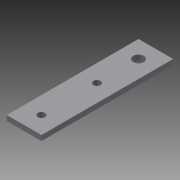
# Autodesk Inventor part: servo catch front c
Saved by Autodesk Inventor 2015 (Build 190159000, 159)
## iProperties
Created: 2015-06-24
Part Number: servo catch front c
Material: 一般
Document SubType Name: Modeling
Designer: kenta
Density: 1 g/cm^3
Appearance: 既定
Author: kenta
Autodesk Inventor part; units mm, degrees
ref_plane "YZ Plane" through (0, 0, 0) normal (1, 0, 0) x (0, 1, 0)
ref_plane "XZ Plane" through (0, 0, 0) normal (0, 1, 0) x (-1, 0, 0)
ref_plane "XY Plane" through (0, 0, 0) normal (0, 0, 1) x (1, 0, 0)
sketch "スケッチ1" plane through (0, 0, 0) normal (0, 0, 1) x (1, 0, 0)
  line L0 (-5, 19) -> (5, 19)
  line L1 (5, 19) -> (5, -19)
  line L2 (5, -19) -> (-5, -19)
  line L3 (-5, -19) -> (-5, 19)
  line L4 (-5, 19) -> (5, -19) construction
  line L5 (5, 19) -> (-5, -19) construction
  point P0 (0, 0)
  dimension "d0" = 10
  dimension "d1" = 38
  constraints: 12 end point, 2 midpoint, 2 parallel, 1 horizontal, 1 perpendicular
  measures "d0" distance of L1.end L2.end
  measures "d1" distance of L0.end L1.end
extrude "押し出し1" add sketch "スケッチ1" along normal blind 1.5
sketch "スケッチ2" plane through (0, 0, 1.5) normal (0, 0, 1) x (1, 0, 0)
  line L0 (5, 19) -> (-5, 19) projected
  line L1 (5, -19) -> (5, 19) projected
  line L2 (-5, -19) -> (5, -19) projected
  point P0 (0, 0)
  point P1 (0, -14)
  point P2 (0, 2)
  dimension "d6" = 5
  dimension "d7" = 5
  dimension "d8" = 16
  measures "d6" distance from line of point (0, -14) L2
  measures "d7" distance from line of point (0, -14) L1
  measures "d8" distance of point (0, 2) point (0, -14)
hole "穴1" at (0, -14, 1.5) at (0, 2, 1.5) direction (0, 0, -1) diameter 2.1 end through all
sketch "スケッチ3" plane through (0, 0, 1.5) normal (0, 0, 1) x (1, 0, 0)
  line L0 (5, 19) -> (-5, 19) projected
  line L1 (5, -19) -> (5, 19) projected
  point P0 (0, 0)
  point P1 (0, 14)
  dimension "d16" = 5
  dimension "d17" = 5
  measures "d16" distance from line of point (0, 14) L0
  measures "d17" distance from line of point (0, 14) L1
hole "穴2" at (0, 14, 1.5) direction (0, 0, -1) diameter 3.1 end through all
